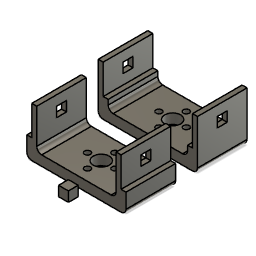
LeArm Bracket (Autodesk Fusion 360 design; units mm, degrees)
Autodesk Fusion 360 part; units mm, degrees
sketch "Sketch1" plane through (0, 0, 0) normal (0, 1, 0) x (1, 0, 0)
  line L0 (-25, 50) -> (25, 50)
  line L1 (25, 50) -> (25, -15)
  line L2 (25, -15) -> (-25, -15)
  line L3 (-25, -15) -> (-25, 50)
  line L4 (-20, 45) -> (20, 45)
  line L5 (20, 45) -> (20, -10)
  line L6 (20, -10) -> (-20, -10)
  line L7 (-20, -10) -> (-20, 45)
  constraint horizontal L0
  constraint vertical L1
  constraint horizontal L2
  constraint vertical L3
  constraint horizontal L4
  constraint vertical L5
  constraint horizontal L6
  constraint vertical L7
extrude "Extrude1" add sketch "Sketch1" along normal blind 25 makes body 1
move_body "Move1" bodies 1 to x (1, 0, 0) y (0, 0, -1) z (0, 1, 0) at (0, 50, -50)
fillet "Fillet1" radius 2.5 4 edges at (25, 65, -62.5) (-25, 65, -62.5) (-25, 0, -62.5) (25, 0, -62.5) on bodies 1
fillet "Fillet2" radius 2.5 4 edges at (-20, 5, -62.5) (-20, 60, -62.5) (20, 60, -62.5) (20, 5, -62.5) on bodies 1
sketch "Sketch2" plane through (0, 5, 0) normal (0, 1, 0) x (-1, 0, 0)
  line L0 (-17.5, -50) -> (-17.5, -75)
  line L1 (-17.5, -75) -> (17.5, -75)
  line L2 (17.5, -75) -> (17.5, -50)
  line L3 (17.5, -50) -> (-17.5, -50)
  circle A0 centre (0, -62.5) radius 4
  dimension "d8" = 8
  measures "d8" diameter of A0
extrude "Extrude2" cut sketch "Sketch2" against normal blind 17 contours A0 bodies 1
sketch "Sketch3" plane through (0, 5, 0) normal (0, 1, 0) x (-1, 0, 0)
  circle A0 centre (0, -62.5) radius 4
  line L0 (-17.5, -50) -> (-17.5, -75)
  line L1 (-17.5, -75) -> (17.5, -75)
  line L2 (17.5, -75) -> (17.5, -50)
  line L3 (17.5, -50) -> (-17.5, -50)
  circle A1 centre (0, -55.6) radius 1.5
  circle A2 centre (0, -69.4) radius 1.5
  circle A3 centre (-6.9, -62.5) radius 1.5
  circle A4 centre (6.9, -62.5) radius 1.5
extrude "Extrude3" cut sketch "Sketch3" against normal blind 11 contours A1 | A2 | A3 | A4 bodies 1
sketch "Sketch4" plane through (0, 0, -50) normal (0, 0, 1) x (1, 0, 0)
  arc A0 (20, 57.5) -> (17.5, 60) centre (17.5, 57.5) ccw
  line L0 (20, 57.5) -> (20, 7.5)
  arc A1 (17.5, 5) -> (20, 7.5) centre (17.5, 7.5) ccw
  line L1 (17.5, 5) -> (-17.5, 5)
  arc A2 (-20, 7.5) -> (-17.5, 5) centre (-17.5, 7.5) ccw
  line L2 (-20, 7.5) -> (-20, 57.5)
  arc A3 (-17.5, 60) -> (-20, 57.5) centre (-17.5, 57.5) ccw
  line L3 (-17.5, 60) -> (17.5, 60)
  arc A4 (22.5, 0) -> (25, 2.5) centre (22.5, 2.5) ccw
  line L4 (25, 2.5) -> (25, 62.5)
  arc A5 (25, 62.5) -> (22.5, 65) centre (22.5, 62.5) ccw
  line L5 (22.5, 65) -> (-22.5, 65)
  arc A6 (-22.5, 65) -> (-25, 62.5) centre (-22.5, 62.5) ccw
  line L6 (-25, 62.5) -> (-25, 2.5)
  arc A7 (-25, 2.5) -> (-22.5, 0) centre (-22.5, 2.5) ccw
  line L7 (-22.5, 0) -> (22.5, 0)
  line L8 (25, 25) -> (-25, 25)
  constraint coincident L6 L8.end
  constraint perpendicular L6 L8
  constraint coincident L4 L8.start
extrude "Extrude4" cut sketch "Sketch4" against normal blind 54 contours A0 L0 L2 A3 L3 L4 A5 L5 A6 L6 L8 bodies 1
copy_body "CopyPasteBodies1" bodies 1 makes body 2
move_body "Move2" bodies 2 to x (1, 0, 0) y (0, 1, 0) z (0, 0, 1) at (0, 0, 36)
sketch "Sketch5" plane through (0, 25, 0) normal (0, 1, 0) x (-1, 0, 0)
  line L0 (-25, -75) -> (-20, -75)
  line L1 (-20, -75) -> (-20, -50)
  line L2 (-20, -50) -> (-25, -50)
  line L3 (-25, -50) -> (-25, -75)
  line L4 (22.5, -75) -> (20, -75)
  line L5 (20, -75) -> (20, -50)
  line L6 (20, -50) -> (22.5, -50)
  line L7 (22.5, -50) -> (22.5, -75)
  line L8 (-22.5, -75) -> (-20, -75)
  line L9 (-20, -75) -> (-20, -50)
  line L10 (-20, -50) -> (-22.5, -50)
  line L11 (-22.5, -50) -> (-22.5, -75)
  constraint midpoint L0 L8.start
  constraint horizontal L4
  constraint vertical L5
  constraint horizontal L6
  constraint vertical L7
  constraint horizontal L8
  constraint vertical L9
  constraint horizontal L10
  constraint vertical L11
  constraint coincident L1.end L2.start
sketch "Sketch6" plane through (0, 25, 0) normal (0, 1, 0) x (-1, 0, 0)
  line L0 (20, -39) -> (25, -39)
  line L1 (25, -39) -> (25, -14)
  line L2 (25, -14) -> (20, -14)
  line L3 (20, -14) -> (20, -39)
  line L4 (22.5, -39) -> (25, -39)
  line L5 (25, -39) -> (25, -14)
  line L6 (25, -14) -> (22.5, -14)
  line L7 (22.5, -14) -> (22.5, -39)
  line L8 (-22.5, -39) -> (-25, -39)
  line L9 (-25, -39) -> (-25, -14)
  line L10 (-25, -14) -> (-22.5, -14)
  line L11 (-22.5, -14) -> (-22.5, -39)
  constraint horizontal L4
  constraint vertical L5
  constraint horizontal L6
  constraint vertical L7
  constraint coincident L1.end L2.start
  constraint midpoint L0 L4.start
  constraint horizontal L8
  constraint vertical L9
  constraint horizontal L10
  constraint vertical L11
extrude "Extrude5" cut sketch "Sketch5" against normal blind 15 contours L0 L1 L2 L8 L9 L10 L11 | L4 L5 L6 L7 bodies 1
extrude "Extrude6" cut sketch "Sketch6" against normal blind 15 contours L0 L1 L2 L4 L5 L6 L7 | L8 L9 L10 L11 bodies 2
sketch "Sketch7" plane through (22.5, 0, 0) normal (1, 0, 0) x (0, 0, -1)
  line L0 (39, 25) -> (14, 25)
  line L1 (14, 25) -> (14, 10)
  line L2 (14, 10) -> (39, 10)
  line L3 (39, 10) -> (39, 25)
  line L4 (29, 15) -> (24, 15)
  line L5 (24, 15) -> (24, 20)
  line L6 (24, 20) -> (29, 20)
  line L7 (29, 20) -> (29, 15)
  line L8 (29, 15) -> (24, 20) construction
  line L9 (24, 15) -> (29, 20) construction
  point P0 (26.5, 17.5)
  constraint horizontal L4
  constraint perpendicular L4 L5
  constraint parallel L4 L6
  constraint parallel L5 L7
  constraint coincident L8 P0
  constraint coincident L9 P0
sketch "Sketch8" plane through (25, 0, 0) normal (1, 0, 0) x (0, 0, -1)
  line L0 (75, 25) -> (50, 25)
  line L1 (50, 25) -> (50, 2.5)
  line L2 (50, 2.5) -> (75, 2.5)
  line L3 (75, 2.5) -> (75, 25)
  line L4 (65, 15) -> (60, 15)
  line L5 (60, 15) -> (60, 20)
  line L6 (60, 20) -> (65, 20)
  line L7 (65, 20) -> (65, 15)
  line L8 (65, 15) -> (60, 20) construction
  line L9 (60, 15) -> (65, 20) construction
  point P0 (62.5, 17.5)
  dimension "d23" = 5
  constraint horizontal L4
  constraint perpendicular L4 L5
  constraint parallel L4 L6
  constraint parallel L5 L7
  constraint coincident L8 P0
  constraint coincident L9 P0
  measures "d23" distance of L4.end L5.end
extrude "Extrude7" cut sketch "Sketch7" against normal blind 71 contours L4 L5 L6 L7 bodies 2
extrude "Extrude8" cut sketch "Sketch8" against normal blind 55 contours L4 L5 L6 L7 bodies 1
sketch "Sketch9" plane through (0, 0, 0) normal (0, 1, 0) x (1, 0, 0)
  line L0 (0, 5) -> (4.95, 5)
  line L1 (4.95, 5) -> (4.95, 9.95)
  line L2 (4.95, 9.95) -> (0, 9.95)
  line L3 (0, 9.95) -> (0, 5)
  dimension "d28" = 4.95
  dimension "d29" = 4.95
  constraint horizontal L0
  constraint vertical L1
  constraint horizontal L2
  constraint vertical L3
  measures "d28" distance of L0.start L0.end
  measures "d29" distance of L0.start L2.end
extrude "Extrude9" add sketch "Sketch9" along normal blind 5 separate body makes body 3
named bodies: "Bracket 1", "Bracket 2", "Pin"
